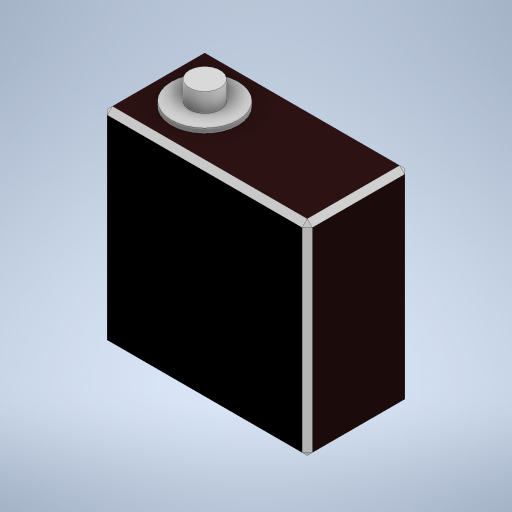
# Autodesk Inventor part: DualServo
Saved by Autodesk Inventor 2023 (Build 270158000, 158)
## iProperties
Created: 2023-01-19
Part Number: DualServo
Material: Generic
Document SubType Name: Modeling
Designer: denyh
Density: 1 g/cm^3
Appearance: Default
Author: denyh
Autodesk Inventor part; units mm, degrees
ref_plane "YZ Plane" through (0, 0, 0) normal (1, 0, 0) x (0, 1, 0)
ref_plane "XZ Plane" through (0, 0, 0) normal (0, 1, 0) x (-1, 0, 0)
ref_plane "XY Plane" through (0, 0, 0) normal (0, 0, 1) x (1, 0, 0)
sketch "Sketch1" plane through (0, 0, 0) normal (0, 0, 1) x (1, 0, 0)
  line L0 (0, 0) -> (40, 0)
  line L1 (40, 0) -> (40, 40)
  line L2 (40, 40) -> (0, 40)
  line L3 (0, 40) -> (0, 0)
  dimension "d0" = 40
  dimension "d1" = 40
  constraints: 8 end point, 2 parallel, 1 horizontal, 1 perpendicular
  measures "d0" distance of L2.end L1.end
  measures "d1" distance of L0.end L1.end
extrude "Extrusion1" add sketch "Sketch1" along normal blind 20
chamfer "Chamfer1" distance 1 angle 45 12 edges at (20, 40, 20) (20, 40, 0) (40, 40, 10) (40, 20, 20) (40, 20, 0) (40, 0, 10) (20, 0, 20) (0, 20, 20) (0, 40, 10) (0, 20, 0) (0, 0, 10) (20, 0, 0)
sketch "Sketch2" plane through (1, 40, 1) normal (0, 1, 0) x (1, 0, 0)
  line L0 (-1, -18) -> (-1, 0) projected
  line L1 (-1, -9) -> (9, -9)
  circle A0 centre (9, -9) radius 3
  point P0 (-1, 1)
  dimension "d7" = 10
  dimension "d8" = 6
  constraints: 2 end point, 1 centre point, 1 coincident, 1 horizontal, 1 midpoint
  measures "d7" distance of L1.start L1.end
  measures "d8" diameter of A0
extrude "Extrusion2" add sketch "Sketch2" along normal blind 4.6
sketch "Sketch3" plane through (1, 40, 1) normal (0, 1, 0) x (1, 0, 0)
  circle A0 centre (9, -9) radius 3 projected
  circle A1 centre (9, -9) radius 6.5
  point P0 (-1, 1)
  dimension "d11" = 13
  constraints: 1 centre point, 1 coincident
  measures "d11" diameter of A1
extrude "Extrusion3" add sketch "Sketch3" along normal blind 0.9
sketch "Sketch5" plane through (1, 0, 19) normal (0, -1, 0) x (1, 0, 0)
  line L0 (-1, 0) -> (-1, -18) projected
  line L1 (-1, -9) -> (9, -9)
  circle A0 centre (9, -9) radius 3
  point P0 (-1, -19)
  dimension "d14" = 10
  constraints: 2 end point, 1 centre point, 1 coincident, 1 horizontal, 1 midpoint
  measures "d14" distance of L1.start L1.end
extrude "Extrusion4" add sketch "Sketch5" along normal blind 5.2
sketch "Sketch6" plane through (1, 0, 19) normal (0, -1, 0) x (1, 0, 0)
  circle A0 centre (9, -9) radius 3 projected
  circle A1 centre (9, -9) radius 6.5
  point P0 (-1, -19)
  dimension "d17" = 13
  constraints: 1 centre point, 1 coincident
  measures "d17" diameter of A1
extrude "Extrusion5" add sketch "Sketch6" along normal blind 1.5 contours A0 | A1
body "Solid1"
